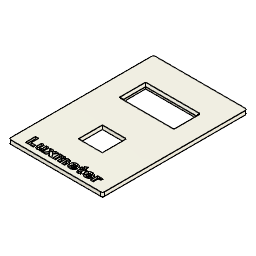
Luxmeter_Cover_V2.0 (Autodesk Fusion 360 design; units mm, degrees)
Autodesk Fusion 360 part; units mm, degrees
sketch "Sketch1" plane through (0, 0, 0) normal (0, 0, 1) x (1, 0, 0)
  line L0 (0, 74) -> (48, 74)
  line L1 (48, 74) -> (48, 0)
  line L2 (48, 0) -> (0, 0)
  line L3 (0, 0) -> (0, 74)
  dimension "d1" = 48
  dimension "d2" = 74
  constraint horizontal L0
  constraint vertical L1
  constraint horizontal L2
  constraint vertical L3
  measures "d1" distance of L0.start L0.end
  measures "d2" distance of L0.start L2.end
extrude "Extrude1" add sketch "Sketch1" against normal blind 2
sketch "Sketch2" plane through (0, 0, -2) normal (0, 0, -1) x (1, 0, 0)
  line L0 (46.75, -72.75) -> (1.25, -72.75)
  line L1 (1.25, -72.75) -> (1.25, -1.25)
  line L2 (1.25, -1.25) -> (46.75, -1.25)
  line L3 (46.75, -1.25) -> (46.75, -72.75)
  dimension "d5" = 45.5
  dimension "d6" = 71.5
  constraint horizontal L0
  constraint vertical L1
  constraint horizontal L2
  constraint vertical L3
  measures "d5" distance of L0.start L0.end
  measures "d6" distance of L0.start L2.end
sketch "Sketch3" plane through (0, 0, -2) normal (0, 0, -1) x (1, 0, 0)
  line L0 (46.5, -72.5) -> (1.5, -72.5)
  line L1 (1.5, -72.5) -> (1.5, -1.5)
  line L2 (1.5, -1.5) -> (46.5, -1.5)
  line L3 (46.5, -1.5) -> (46.5, -72.5)
  dimension "d7" = 45
  dimension "d8" = 71
  constraint horizontal L0
  constraint vertical L1
  constraint horizontal L2
  constraint vertical L3
  measures "d7" distance of L0.start L0.end
  measures "d8" distance of L0.start L2.end
extrude "Extrude2" add sketch "Sketch3" along normal blind 1.5 thin wall 1.5 inside
sketch "Sketch4" plane through (0, 0, 0) normal (0, 0, 1) x (-1, 0, 0)
  line L0 (-11, -59) -> (-37, -59)
  line L1 (-37, -59) -> (-37, -47.5)
  line L2 (-37, -47.5) -> (-11, -47.5)
  line L3 (-11, -47.5) -> (-11, -59)
  dimension "d12" = 26
  dimension "d13" = 11.5
  constraint horizontal L0
  constraint vertical L1
  constraint horizontal L2
  constraint vertical L3
  measures "d12" distance of L0.start L0.end
  measures "d13" distance of L0.start L2.end
sketch "Sketch5" plane through (0, 0, 0) normal (0, 0, 1) x (-1, 0, 0)
  line L0 (-17.9, -30) -> (-30.1, -30)
  line L1 (-30.1, -30) -> (-30.1, -17.8)
  line L2 (-30.1, -17.8) -> (-17.9, -17.8)
  line L3 (-17.9, -17.8) -> (-17.9, -30)
  dimension "d14" = 12.2
  dimension "d15" = 12.2
  constraint horizontal L0
  constraint vertical L1
  constraint horizontal L2
  constraint vertical L3
  measures "d14" distance of L0.start L0.end
  measures "d15" distance of L0.start L2.end
extrude "Extrude3" cut sketch "Sketch4" against normal blind 2
extrude "Extrude4" cut sketch "Sketch5" against normal blind 2
fillet "Fillet1" radius 1 4 edges at (24, 59, 0) (37, 53.25, 0) (24, 47.5, 0) (11, 53.25, 0)
fillet "Fillet2" radius 1 4 edges at (48, 74, -1) (0, 74, -1) (0, 0, -1) (48, 0, -1)
sketch "Sketch6" plane through (0, 0, 0) normal (0, 0, 1) x (-1, 0, 0)
  line L0 (-1.4595, -2.783) -> (-46.5222, -2.6038) construction
  line L1 (-46.5222, -2.6038) -> (-46.5405, -7.217) construction
  line L2 (-46.5405, -7.217) -> (-1.4778, -7.3962) construction
  line L3 (-1.4778, -7.3962) -> (-1.4595, -2.783) construction
  dimension "d24" = 5
  text T0 "Luxmeter" font "Arial Black" height 5 align centre bottom in box 45.0631 x 4.6133 at (-1.4595, -2.783) x (-0.999992, 0.003977) y (-0.003977, -0.999992) spacing 1
extrude "Extrude5" cut sketch "Sketch6" against normal blind 1 text T0
equation "d25 = 'Luxmeter'"
